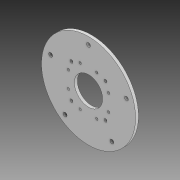
# Autodesk Inventor part: J0_motorbracket
Saved by Autodesk Inventor 2020 (Build 240168000, 168)
## iProperties
Created: 2021-03-20
Part Number: J0_motorbracket
Material: Generic
Document SubType Name: Modeling
Designer: DDeGo
Density: 1 g/cm^3
Appearance: Default
Author: DDeGo
Autodesk Inventor part; units mm, degrees
ref_plane "YZ Plane" through (0, 0, 0) normal (1, 0, 0) x (0, 1, 0)
ref_plane "XZ Plane" through (0, 0, 0) normal (0, 1, 0) x (-1, 0, 0)
ref_plane "XY Plane" through (0, 0, 0) normal (0, 0, 1) x (1, 0, 0)
sketch "Sketch1" plane through (0, 0, 0) normal (0, 0, 1) x (1, 0, 0)
  circle A0 centre (0, 55) radius 2.65
  arc A1 (65, 0) -> (-65, 0) centre (0, 0) ccw
  line L0 (-65, 0) -> (-65, -80)
  line L1 (-65, -80) -> (65, -80)
  line L2 (65, -80) -> (65, 0)
  circle A2 centre (0, 0) radius 47.5 construction
  circle A3 centre (0, 0) radius 55 construction
  line L3 (0, 55) -> (0, 0) construction
  circle A4 centre (-52.3081, 16.9959) radius 2.65
  circle A5 centre (-32.3282, -44.4959) radius 2.65
  circle A6 centre (32.3282, -44.4959) radius 2.65
  circle A7 centre (52.3081, 16.9959) radius 2.65
  dimension "d23" = 110
  dimension "d24" = 95
  dimension "d25" = 65
  dimension "d26" = 80
  dimension "d27" = 5.3
  dimension "d30" = 360
  constraints: 8 end point, 7 centre point, 3 coincident, 3 vertical, 2 point on circle, 2 tangent, 1 horizontal, 1 vertical alignment, 13 other
  measures "d24" diameter of A2
  measures "d25" radius of A1
  measures "d26" distance from line of L1 point (0, 0)
  measures "d27" diameter of A0
extrude "Extrusion1" add sketch "Sketch1" along normal blind 4
sketch "Sketch2" plane through (0, 0, 4) normal (0, 0, 1) x (1, 0, 0)
  circle A0 centre (0, 0) radius 19.5
  line L0 (-23.5, -23.5) -> (23.5, -23.5) construction
  line L1 (23.5, -23.5) -> (23.5, 23.5) construction
  line L2 (23.5, 23.5) -> (-23.5, 23.5) construction
  line L3 (-23.5, 23.5) -> (-23.5, -23.5) construction
  line L4 (-23.5, -23.5) -> (23.5, 23.5) construction
  line L5 (23.5, -23.5) -> (-23.5, 23.5) construction
  circle A1 centre (-23.5, 23.5) radius 2
  circle A2 centre (23.5, 23.5) radius 2
  circle A3 centre (23.5, -23.5) radius 2
  circle A4 centre (-23.5, -23.5) radius 2
  dimension "d2" = 39
  dimension "d3" = 47
  dimension "d4" = 4
  constraints: 12 end point, 5 centre point, 5 coincident, 3 equal radius, 2 midpoint, 2 parallel, 2 perpendicular, 1 horizontal
  measures "d2" diameter of A0
  measures "d3" distance of L2.end L0.start
  measures "d4" diameter of A1
extrude "Extrusion2" cut sketch "Sketch2" against normal through all
sketch "Sketch3" plane through (0, 0, 4) normal (0, 0, 1) x (1, 0, 0)
  arc A0 (65, 0) -> (-65, 0) centre (0, 0) ccw projected
  circle A1 centre (0, 0) radius 65
  circle A2 centre (0, 0) radius 147.6285
  point P0 (65, 0)
  constraints: 2 coincident, 1 centre point, 3 other
extrude "Extrusion3" cut sketch "Sketch3" against normal through all
sketch "Sketch4" plane through (0, 0, 4) normal (0, 0, 1) x (1, 0, 0)
  circle A0 centre (0, 0) radius 30 construction
  circle A1 centre (-27.7164, 11.4805) radius 1.6
  line L0 (-27.7164, 11.4805) -> (0, 0) construction
  line L1 (-27.7164, -11.4805) -> (0, 0) construction
  circle A2 centre (-27.7164, -11.4805) radius 1.6
  line L2 (-11.4805, -27.7164) -> (0, 0) construction
  circle A3 centre (-11.4805, -27.7164) radius 1.6
  line L3 (11.4805, -27.7164) -> (0, 0) construction
  circle A4 centre (11.4805, -27.7164) radius 1.6
  line L4 (27.7164, -11.4805) -> (0, 0) construction
  circle A5 centre (27.7164, -11.4805) radius 1.6
  line L5 (27.7164, 11.4805) -> (0, 0) construction
  circle A6 centre (27.7164, 11.4805) radius 1.6
  line L6 (11.4805, 27.7164) -> (0, 0) construction
  circle A7 centre (11.4805, 27.7164) radius 1.6
  line L7 (-11.4805, 27.7164) -> (0, 0) construction
  circle A8 centre (-11.4805, 27.7164) radius 1.6
  line L8 (0, 0) -> (-27.7164, 0) construction
  line L9 (-27.7164, 0) -> (-27.7164, 11.4805) construction
  line L10 (-27.7164, 0) -> (-27.7164, -11.4805) construction
  dimension "d9" = 60
  dimension "d10" = 3.2
  dimension "d13" = 360
  constraints: 22 end point, 8 centre point, 1 coincident, 1 horizontal, 1 perpendicular, 1 vertical, 36 other
  measures "d10" diameter of A1
extrude "Extrusion4" cut sketch "Sketch4" against normal through all
body "Solid1"
